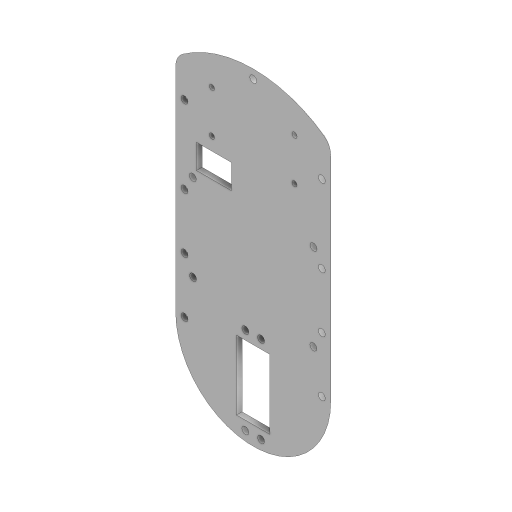
# Autodesk Inventor part: baseboard
Saved by Autodesk Inventor 2024 (Build 280153000, 153)
## iProperties
Created: 2024-07-11
Part Number: baseboard
Material: Generic
Document SubType Name: Modeling
Designer: chris
Density: 1 g/cm^3
Appearance: Default
Author: chris
Autodesk Inventor part; units mm, degrees
ref_plane "YZ Plane" through (0, 0, 0) normal (1, 0, 0) x (0, 1, 0)
ref_plane "XZ Plane" through (0, 0, 0) normal (0, 1, 0) x (-1, 0, 0)
ref_plane "XY Plane" through (0, 0, 0) normal (0, 0, 1) x (1, 0, 0)
sketch "Sketch1" plane through (0, 0, 0) normal (0, 0, 1) x (1, 0, 0)
  arc A0 (-3.0019, -15.825) -> (-5.9981, -15.825) centre (-4.5, -14.5) ccw
  circle A1 centre (-4.5, -14.5) radius 2
  line L0 (0, -9.42) -> (0, -13.0717)
  line L1 (-4.5, -14.5) -> (-4.5, -9.42)
  line L2 (9.58, -9.42) -> (0, -9.42)
  line L3 (-9.573, -9.42) -> (0, -9.42)
  circle A2 centre (0, 0) radius 2
  line L4 (-20.6375, 0) -> (0, 0)
  line L5 (9.58, 30.2602) -> (9.58, -9.42)
  line L6 (-9.573, 30.2602) -> (-9.573, -9.42)
  line L7 (4.5, 30.2602) -> (9.58, 30.2602)
  line L8 (-4.493, 30.2602) -> (-9.573, 30.2602)
  circle A3 centre (0, 0) radius 2
  line L9 (4.5, 30.2602) -> (-4.493, 30.2602)
  line L10 (4.507, 35.3402) -> (4.5, 30.2602)
  arc A4 (6.0051, 34.0152) -> (3.0089, 34.0152) centre (4.507, 35.3402) ccw
  circle A5 centre (4.507, 35.3402) radius 2
  arc A6 (-2.9949, 34.0152) -> (-5.9911, 34.0152) centre (-4.493, 35.3402) ccw
  circle A7 centre (-4.493, 35.3402) radius 2
  line L11 (-4.493, 35.3402) -> (-4.493, 30.2602)
  circle A8 centre (4.5, -14.5) radius 2
  arc A9 (5.9981, -15.825) -> (3.0019, -15.825) centre (4.5, -14.5) ccw
  line L12 (-32.4965, 44.5477) -> (32.5035, 44.5477)
  line L13 (-32.4965, 114.5477) -> (-32.4965, 100.5477)
  line L14 (-32.4965, 44.5477) -> (-32.4965, 114.5477)
  line L15 (32.5035, 44.5477) -> (32.5035, 114.5477)
  line L16 (-32.4965, 114.5477) -> (32.5035, 114.5477)
  line L17 (32.5035, 114.5477) -> (32.5035, 44.5477)
  line L18 (32.5035, 44.5477) -> (-32.4965, 44.5477)
  line L19 (-32.4965, 100.5477) -> (-12.4965, 100.5477)
  line L20 (-12.4965, 114.5477) -> (-12.4965, 100.5477)
  line L21 (-32.4965, 100.5477) -> (-12.4965, 100.5477)
  line L22 (-12.4965, 100.5477) -> (-12.4965, 114.5477)
  line L23 (-12.4965, 114.5477) -> (-32.4965, 114.5477)
  line L24 (0.0035, 44.5477) -> (0.0035, 15.9727)
  line L25 (0.0035, 30.2602) -> (0.0035, 18.2859)
  line L26 (0.0035, 30.2602) -> (13.164, 30.2602)
  line L27 (-23.1486, 122.8027) -> (23.1556, 122.8027)
  line L28 (0.0035, 114.5477) -> (2, 109.97)
  line L29 (0.0035, 114.5477) -> (0.0035, 122.8027)
  circle A10 centre (0.0035, 24.273) radius 44.45
  line L30 (-44.4465, 24.273) -> (-44.4465, 151.273)
  line L31 (-44.4465, 151.273) -> (44.4535, 151.273)
  line L32 (44.4535, 151.273) -> (44.4535, 24.273)
  arc A11 (44.4535, 151.273) -> (-44.4465, 151.273) centre (0.0035, 97.3915) ccw
  line L33 (-32.4965, 100.5477) -> (-34.5965, 100.5477)
  line L34 (-32.4965, 44.5477) -> (-32.4965, 54.5972)
  line L35 (-32.4965, 54.5972) -> (-34.5965, 54.5972)
  line L36 (0.0035, 97.3915) -> (0.0035, 87.773)
  line L37 (-44.4465, 24.273) -> (-39.3665, 24.273)
  circle A12 centre (-39.3665, 24.273) radius 2
  line L38 (-44.4465, 151.273) -> (-44.4465, 132.223)
  line L39 (-44.4465, 132.223) -> (-39.3665, 132.223)
  circle A13 centre (-39.3665, 132.223) radius 2
  line L40 (-44.4465, 87.773) -> (-39.3665, 87.773)
  circle A14 centre (-39.3665, 87.773) radius 2
  line L41 (0.0035, 167.2415) -> (0.0035, 162.1615)
  circle A15 centre (0.0035, 162.1615) radius 2
  line L42 (-44.4465, 24.273) -> (-44.4465, 87.773)
  line L43 (-44.4465, 56.023) -> (-39.3665, 56.023)
  circle A16 centre (-39.3665, 56.023) radius 2
  line L44 (-32.4965, 44.5477) -> (-32.4965, 46.5477)
  line L45 (-32.4965, 46.5477) -> (-34.4965, 46.5477)
  circle A17 centre (-34.4965, 46.5477) radius 2
  circle A18 centre (39.3735, 24.273) radius 2
  circle A19 centre (39.3735, 132.223) radius 2
  circle A20 centre (39.3735, 87.773) radius 2
  circle A21 centre (39.3735, 56.023) radius 2
  circle A22 centre (34.5035, 46.5477) radius 2
  line L46 (-34.5965, 100.5477) -> (-34.5965, 96.1027)
  circle A23 centre (-34.5965, 96.1027) radius 2
  circle A24 centre (34.6035, 96.1027) radius 2
  line L47 (-39.3665, 132.223) -> (-39.3665, 119.523)
  circle A25 centre (-39.3665, 119.523) radius 2
  circle A26 centre (39.3735, 119.523) radius 2
  line L48 (-23.1486, 145.5103) -> (23.1556, 145.5103)
  line L49 (0.0035, 145.5103) -> (0.0035, 122.8027)
  line L50 (0.0035, 134.1565) -> (-9.573, 134.1565)
  line L51 (-28.6515, 134.1565) -> (-23.6515, 134.1565)
  line L52 (-23.6515, 134.1565) -> (-23.6515, 146.2515)
  line L53 (-23.6515, 134.1565) -> (-23.6515, 122.0615)
  line L54 (-23.6515, 134.1565) -> (23.6585, 134.1565)
  circle A27 centre (-23.6515, 146.2515) radius 1.5
  circle A28 centre (-23.6515, 122.0615) radius 1.5
  line L55 (0.0035, 134.1565) -> (0.0035, 148.8537)
  circle A29 centre (23.6585, 146.2515) radius 1.5
  circle A30 centre (23.6585, 122.0615) radius 1.5
  point P0 (0.0035, 58.0477)
  point P1 (-3.0019, -15.825)
  point P2 (-5.9981, -15.825)
  point P3 (3.0089, 34.0152)
  point P4 (6.0051, 34.0152)
  dimension "d3" = 28.575
  dimension "d7" = 8.255
  dimension "d8" = 88.9
  dimension "d9" = 127
  dimension "d10" = 88.9
  dimension "d11" = 69.85
  dimension "d15" = 2.1
  dimension "d17" = 2.1
  dimension "d19" = 5.08
  dimension "d20" = 4
  dimension "d21" = 19.05
  dimension "d22" = 5.08
  dimension "d23" = 4
  dimension "d24" = 5.08
  dimension "d25" = 4
  dimension "d26" = 5.08
  dimension "d27" = 4
  dimension "d28" = 5.08
  dimension "d29" = 4
  dimension "d30" = 2
  dimension "d31" = 2
  dimension "d32" = 4
  dimension "d33" = 4.445
  dimension "d34" = 4
  dimension "d35" = 12.7
  dimension "d36" = 4
  dimension "d38" = 5
  dimension "d39" = 12.095
  dimension "d40" = 47.31
  dimension "d41" = 3
  dimension "d42" = 3
  constraints: 112 end point, 31 centre point, 16 coincident, 14 point on circle, 12 perpendicular, 10 midpoint, 10 symmetric about line, 10 vertical, 8 horizontal, 4 point on line, 3 collinear, 1 parallel, 9 other
  measures "d3" distance of L24.start L24.end
  measures "d7" distance of L28.start L29.end
  measures "d8" diameter of A10
  measures "d9" distance of L30.start L30.end
  measures "d10" distance of L30.end L31.end
  measures "d11" radius of A11
  measures "d15" distance of L13.end L33.end
  measures "d17" distance of L34.end L35.end
  measures "d19" distance of L30.start L37.end
  measures "d20" diameter of A12
  measures "d21" distance of L30.end L38.end
  measures "d22" distance of L38.end L39.end
  measures "d23" diameter of A13
  measures "d24" distance of L40.start L40.end
  measures "d25" diameter of A14
  measures "d26" distance of L41.start L41.end
  measures "d27" diameter of A15
  measures "d28" distance of L43.start L43.end
  measures "d29" diameter of A16
  measures "d30" distance of L12.start L44.end
  measures "d31" distance of L44.end L45.end
  measures "d32" diameter of A17
  measures "d33" distance of L46.start L46.end
  measures "d34" diameter of A23
  measures "d35" distance of L47.start L47.end
  measures "d36" diameter of A25
  measures "d38" distance of L51.start L54.start
  measures "d39" distance of L54.start L52.end
  measures "d40" distance of L54.start L54.end
  measures "d41" diameter of A27
  measures "d42" diameter of A28
extrude "Extrusion1" add sketch "Sketch1" along normal blind 3.175 contours L14 A10 L15 L12 | L12 L15 A10 L14 | A10 L30 L31 L32 L15 L16 L13 L14 | L14 L19 L20 L16 L15 A10 | L31 A11 | A28 L53 L54 L50 L49 L27 | L50 L54 L52 A27 L48 L49 | A25 | A26
fillet "Fillet1" radius 9.525 2 edges at (-44.4465, 151.273, 1.5875) (44.4535, 151.273, 1.5875)
fillet "Fillet2" radius 9.525 6 edges at (43.3917, 150.9488, 0) (0.0035, 167.2415, 0) (-43.3847, 150.9488, 0) (-44.4465, 85.4257, 0) (0.0035, -20.177, 0) (44.4535, 85.4257, 0)
body "Solid1"
